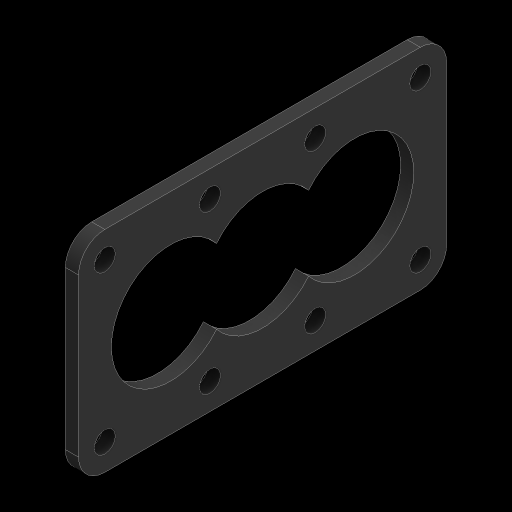
# Autodesk Inventor part: ANS8-5-BK
Saved by Autodesk Inventor 2024 (Build 280153000, 153)
## iProperties
Created: 2023-10-14
Part Number: ANS8-5-BK
Material: Rubber
Document SubType Name: Modeling
Designer: bennk
Mass: 60.2658 g
Surface Area: 278.751 cm^2
Volume: 64.8019 cm^3
Density: 0.93 g/cm^3
Appearance: Rubber - Black
Author: bennk
Autodesk Inventor part; units mm, degrees
ref_plane "YZ Plane" through (0, 0, 0) normal (1, 0, 0) x (0, 1, 0)
ref_plane "XZ Plane" through (0, 0, 0) normal (0, 1, 0) x (-1, 0, 0)
ref_plane "XY Plane" through (0, 0, 0) normal (0, 0, 1) x (1, 0, 0)
sketch "Sketch1" plane through (0, 0, 0) normal (1, 0, 0) x (0, 1, 0)
  line L0 (50.8, -88.9) -> (-50.8, -88.9)
  line L1 (-50.8, -88.9) -> (-50.8, 88.9)
  line L2 (-50.8, 88.9) -> (50.8, 88.9)
  line L3 (50.8, 88.9) -> (50.8, -88.9)
  line L4 (50.8, -88.9) -> (-50.8, 88.9) construction
  line L5 (-50.8, -88.9) -> (50.8, 88.9) construction
  point P0 (0, 0)
  dimension "d0" = 101.6
  dimension "d1" = 177.8
  constraints: 12 end point, 2 midpoint, 2 parallel, 1 horizontal, 1 perpendicular
  measures "d0" distance of L1.end L2.end
  measures "d1" distance of L0.end L1.end
extrude "RECTANGLE" add sketch "Sketch1" along normal blind 6.35
fillet "FILLETS" radius 12.7 4 edges at (3.175, 50.8, 88.9) (3.175, -50.8, 88.9) (3.175, 50.8, -88.9) (3.175, -50.8, -88.9)
sketch "Sketch2" plane through (6.35, 0, 0) normal (1, 0, 0) x (0, 0, -1)
  arc A0 (-88.9, -38.1) -> (-76.2, -50.8) centre (-76.2, -38.1) ccw projected
  point P0 (0, 0)
  constraints: 1 coincident
hole "SMALL HOLE" at (6.35, -38.1, 76.2) direction (-1, 0, 0) diameter 10.16 end through all
pattern_linear "SMALL HOLES" count 4 spacing 50.8 along (0, 0, -1) count 2 spacing 76.2 along (0, 1, 0) of "SMALL HOLE"
sketch "Sketch3" plane through (6.35, 0, 0) normal (1, 0, 0) x (0, 0, -1)
  line L0 (-88.9, 38.1) -> (-88.9, -38.1) projected
  point P0 (0, 0)
  point P1 (-44.45, 0)
  dimension "d25" = 44.45
  dimension "d26" = 0
  measures "d25" distance from line of L0 point (-44.45, 0)
  measures "d26" vertical distance of point (0, 0) point (-44.45, 0)
hole "LARGE HOLE" at (6.35, 0, 44.45) direction (-1, 0, 0) diameter 57.15 end through all
pattern_linear "LARGE HOLES" count 3 spacing 44.45 along (0, 0, -1) of "LARGE HOLE"
body "Solid1"
